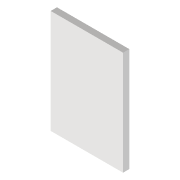
# Autodesk Inventor part: 00_Huawei_P30_Lens_Adapterpcb
Saved by Autodesk Inventor 2022 (Build 260153000, 153)
## iProperties
Created: 2022-12-14
Part Number: 00_Huawei_P30_Lens_Adapterpcb
Material: Generisch
Document SubType Name: Modeling
Designer: diederichbenedict
Density: 1 g/cm^3
Appearance: Vorgabe
Author: diederichbenedict
Autodesk Inventor part; units mm, degrees
ref_plane "YZ Plane" through (0, 0, 0) normal (1, 0, 0) x (0, 1, 0)
ref_plane "XZ Plane" through (0, 0, 0) normal (0, 1, 0) x (-1, 0, 0)
ref_plane "XY Plane" through (0, 0, 0) normal (0, 0, 1) x (1, 0, 0)
sketch "Skizze1" plane through (0, 0, 0) normal (0, 0, 1) x (1, 0, 0)
  line L0 (-9.25, -6.8) -> (-9.25, 6.8) projected
  line L1 (9.25, -6.8) -> (-9.25, -6.8) projected
  line L2 (9.25, 6.8) -> (9.25, -6.8) projected
  line L3 (-9.25, 6.8) -> (9.25, 6.8) projected
  line L4 (12.85, -16.45) -> (-8.15, -16.45)
  line L5 (-8.15, -16.45) -> (-8.15, 8.55)
  line L6 (-8.15, 8.55) -> (12.85, 8.55)
  line L7 (12.85, 8.55) -> (12.85, -16.45)
  point P0 (0, 0)
  dimension "d0" = 21
  dimension "d1" = 25
  dimension "d2" = 3.6
  dimension "d6" = 1.75
  constraints: 8 end point, 2 parallel, 1 horizontal, 1 perpendicular
  measures "d0" distance of L5.end L6.end
  measures "d1" distance of L4.end L5.end
  measures "d2" distance between parallel lines of L7 L2
  measures "d6" distance between parallel lines of L3 L6
extrude "Extrusion1" add sketch "Skizze1" along normal blind 1.5 contours L5 L3 L2 L1 | L1 L2 L3 L5 L6 L7 L4
sketch "Skizze2" plane through (0, 0, 1.5) normal (0, 0, 1) x (1, 0, 0)
  line L0 (9.25, -6.8) -> (-9.25, -6.8) projected
  line L1 (-8.15, -16.45) -> (12.85, -16.45) projected
  line L2 (12.85, -16.45) -> (12.85, 8.55) projected
  line L3 (12.85, 8.55) -> (-8.15, 8.55) projected
  line L4 (-8.15, 8.55) -> (-8.15, -16.45) projected
  line L5 (9.25, 6.8) -> (9.25, -6.8) projected
  line L6 (12.85, -16.45) -> (12.85, 8.55) projected
  line L7 (12.85, 8.55) -> (9.25, 8.55)
  line L8 (9.25, 8.55) -> (9.25, -6.8)
  line L9 (9.25, -6.8) -> (12.85, -6.8)
  line L10 (12.85, -6.8) -> (12.85, 8.55)
  point P0 (0, 0)
  constraints: 8 end point, 2 parallel, 1 horizontal, 1 perpendicular
extrude "Extrusion2" cut sketch "Skizze2" against normal blind 10 contours L5 L8 L3 L2 L9
sketch "Skizze3" plane through (0, 0, 0) normal (0, 0, -1) x (-1, 0, 0)
  line L0 (-9.25, 8.55) -> (-9.25, -6.8) projected
  line L1 (-9.25, -6.8) -> (-12.85, -6.8) projected
  line L2 (-12.85, -16.45) -> (-12.85, -6.8) projected
  line L3 (8.15, -16.45) -> (-12.85, -16.45) projected
  line L4 (8.15, 8.55) -> (8.15, -16.45) projected
  line L5 (-9.25, 8.55) -> (8.15, 8.55) projected
  line L6 (-12.85, -16.45) -> (-9.25, -16.45)
  line L7 (-9.25, -16.45) -> (-9.25, -6.8)
  line L8 (-9.25, -6.8) -> (-12.85, -6.8)
  line L9 (-12.85, -6.8) -> (-12.85, -16.45)
  point P0 (0, 0)
  constraints: 8 end point, 2 parallel, 1 horizontal, 1 perpendicular
extrude "Extrusion3" cut sketch "Skizze3" against normal blind 10 contours L7 L3 L2 L1
